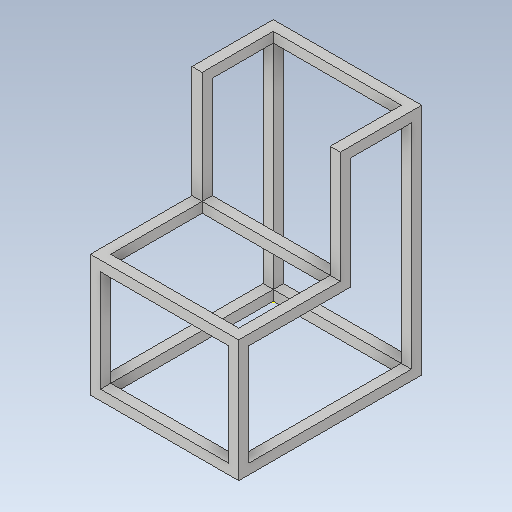
# Autodesk Inventor part: fuel tank housing
Saved by Autodesk Inventor 2020 (Build 240168000, 168)
## iProperties
Created: 2020-10-15
Part Number: fuel tank housing
Material: Generic
Document SubType Name: Modeling
Designer: nabee
Density: 1 g/cm^3
Appearance: Default
Author: nabee
Autodesk Inventor part; units mm, degrees
ref_plane "YZ Plane" through (0, 0, 0) normal (1, 0, 0) x (0, 1, 0)
ref_plane "XZ Plane" through (0, 0, 0) normal (0, 1, 0) x (-1, 0, 0)
ref_plane "XY Plane" through (0, 0, 0) normal (0, 0, 1) x (1, 0, 0)
sketch "Sketch1" plane through (0, 0, 0) normal (0, 0, 1) x (1, 0, 0)
  line L0 (0, 0) -> (220, 0)
  line L1 (220, 0) -> (220, 480)
  line L2 (220, 480) -> (0, 480)
  line L3 (0, 480) -> (0, 0)
  dimension "d0" = 480
  dimension "d1" = 220
  constraints: 8 end point, 2 parallel, 1 horizontal, 1 perpendicular
  measures "d0" distance of L2.end L0.start
  measures "d1" distance of L0.start L0.end
extrude "Extrusion1" add sketch "Sketch1" along normal blind 360
sketch "Sketch2" plane through (0, 480, 0) normal (0, 1, 0) x (1, 0, 0)
  line L0 (220, 0) -> (220, -360) projected
  line L1 (0, 0) -> (220, 0)
  line L2 (220, 0) -> (220, -160)
  line L3 (220, -160) -> (0, -160)
  line L4 (0, -160) -> (0, 0)
  line L5 (20, -20) -> (200, -20)
  line L6 (200, -20) -> (200, -140)
  line L7 (200, -140) -> (20, -140)
  line L8 (20, -140) -> (20, -20)
  line L9 (0, -360) -> (220, -360) projected
  line L10 (0, -160) -> (220, -160)
  line L11 (220, -160) -> (220, -360)
  line L12 (220, -360) -> (0, -360)
  line L13 (0, -360) -> (0, -160)
  dimension "d4" = 160
  dimension "d5" = 20
  dimension "d6" = 20
  dimension "d7" = 20
  dimension "d8" = 20
  constraints: 24 end point, 6 parallel, 3 horizontal, 3 perpendicular, 1 point on line
  measures "d4" distance of L3.end L1.start
  measures "d5" distance between parallel lines of L1 L5
  measures "d6" distance between parallel lines of L4 L8
  measures "d7" distance between parallel lines of L0 L6
  measures "d8" distance between parallel lines of L3 L7
extrude "Extrusion2" cut sketch "Sketch2" against normal blind 220 contours L0 L9 L13 L3
sketch "Sketch3" plane through (220, 0, 0) normal (1, 0, 0) x (0, 0, -1)
  line L0 (-20, 240) -> (-20, 20)
  line L1 (-20, 20) -> (-340, 20)
  line L2 (-340, 20) -> (-340, 240)
  line L3 (-160, 260) -> (-360, 260) projected
  line L4 (-360, 0) -> (-360, 260) projected
  line L5 (0, 0) -> (-360, 0) projected
  line L6 (0, 0) -> (0, 480) projected
  line L7 (-340, 240) -> (-140, 240)
  line L8 (-140, 240) -> (-140, 460)
  line L9 (-140, 460) -> (-20, 460)
  line L10 (-20, 460) -> (-20, 240)
  line L11 (-160, 480) -> (-160, 260) projected
  line L12 (0, 480) -> (-160, 480) projected
  dimension "d12" = 20
  dimension "d13" = 20
  dimension "d14" = 20
  dimension "d16" = 20
  dimension "d17" = 20
  dimension "d18" = 20
  constraints: 14 end point, 2 equal length, 2 perpendicular, 1 horizontal
  measures "d12" distance between parallel lines of L4 L2
  measures "d13" distance between parallel lines of L5 L1
  measures "d14" distance between parallel lines of L6 L0
  measures "d16" distance between parallel lines of L11 L8
  measures "d17" distance between parallel lines of L12 L9
  measures "d18" distance between parallel lines of L3 L7
extrude "Extrusion3" cut sketch "Sketch3" against normal blind 220 contours L0 L1 L2 L7 L8 L9 L10
sketch "Sketch4" plane through (0, 0, 360) normal (0, 0, 1) x (1, 0, 0)
  line L0 (20, 240) -> (200, 240)
  line L1 (200, 240) -> (200, 20)
  line L2 (200, 20) -> (20, 20)
  line L3 (20, 20) -> (20, 240)
  line L4 (220, 260) -> (0, 260) projected
  line L5 (0, 260) -> (0, 0) projected
  line L6 (0, 0) -> (220, 0) projected
  line L7 (220, 0) -> (220, 260) projected
  dimension "d21" = 20
  dimension "d22" = 20
  dimension "d23" = 20
  dimension "d24" = 20
  constraints: 8 end point, 2 parallel, 1 horizontal, 1 perpendicular
  measures "d21" distance between parallel lines of L4 L0
  measures "d22" distance between parallel lines of L5 L3
  measures "d23" distance between parallel lines of L6 L2
  measures "d24" distance between parallel lines of L7 L1
extrude "Extrusion4" cut sketch "Sketch4" against normal blind 600 contours L0 L1 L2 L3
sketch "Sketch5" plane through (0, 0, 0) normal (0, -1, 0) x (1, 0, 0)
  line L0 (200, 20) -> (200, 0) projected
  line L1 (20, 340) -> (200, 340)
  line L2 (200, 340) -> (200, 20)
  line L3 (200, 20) -> (20, 20)
  line L4 (20, 20) -> (20, 340)
  point P0 (0, 0)
  constraints: 8 end point, 2 parallel, 1 horizontal, 1 perpendicular
extrude "Extrusion5" cut sketch "Sketch5" against normal blind 900
sketch "Sketch6" plane through (0, 0, 0) normal (0, 0, -1) x (-1, 0, 0)
  line L0 (-220, 240) -> (-200, 240) projected
  line L1 (-20, 460) -> (-20, 240) projected
  line L2 (-200, 240) -> (-20, 240)
  line L3 (-20, 240) -> (-20, 460)
  line L4 (-20, 460) -> (-200, 460)
  line L5 (-200, 460) -> (-200, 240)
  point P0 (0, 0)
  constraints: 8 end point, 2 parallel, 1 horizontal, 1 perpendicular
extrude "Extrusion6" cut sketch "Sketch6" against normal blind 80
sketch "Sketch7" plane through (20, 260, 160) normal (1, 0, 0) x (0, 0, -1)
  line L0 (20, 200) -> (20, -20) projected
  line L1 (20, -20) -> (0, -20)
  line L2 (0, -20) -> (0, 0)
  line L3 (0, 0) -> (20, 0)
  line L4 (20, 0) -> (20, -20)
  point P0 (160, -260)
  constraints: 8 end point, 2 parallel, 1 horizontal, 1 perpendicular
extrude "Extrusion7" add sketch "Sketch7" along normal blind 180
sketch "Sketch8" plane through (0, 0, 0) normal (0, -1, 0) x (1, 0, 0)
  point P0 (0, 0)
sketch "Sketch9" plane through (220, 0, 0) normal (1, 0, 0) x (0, 0, -1)
  line L0 (-360, 0) -> (-360, 260) projected
  line L1 (-360, 0) -> (-360, 260)
  line L2 (-360, 260) -> (-160, 260)
  line L3 (-160, 480) -> (-20, 480) projected
  line L4 (-160, 260) -> (-160, 480)
  line L5 (-160, 480) -> (0, 480)
  line L6 (0, 480) -> (0, 0)
  line L7 (0, 0) -> (-360, 0)
  constraints: 12 end point, 4 perpendicular, 1 collinear, 1 vertical
extrude "Extrusion8" add sketch "Sketch9" along normal blind 72
sketch "Sketch10" plane through (292, 0, 0) normal (1, 0, 0) x (0, 0, -1)
  line L0 (-340, 20) -> (-340, 240) projected
  line L1 (-340, 240) -> (-340, 20)
  line L2 (-20, 20) -> (-340, 20) projected
  line L3 (-340, 20) -> (-20, 20)
  line L4 (0, 460) -> (-20, 460) projected
  line L5 (-20, 20) -> (-20, 460)
  line L6 (-20, 460) -> (-140, 460)
  line L7 (-140, 240) -> (-340, 240) projected
  line L8 (-140, 460) -> (-140, 240)
  line L9 (-140, 240) -> (-340, 240)
  point P0 (0, 0)
  constraints: 12 end point, 3 perpendicular, 2 collinear, 1 vertical
extrude "Extrusion9" cut sketch "Sketch10" against normal blind 150
sketch "Sketch11" plane through (0, 0, 360) normal (0, 0, 1) x (1, 0, 0)
  line L0 (20, 240) -> (200, 240) projected
  line L1 (292, 20) -> (200, 20) projected
  line L2 (200, 240) -> (272, 240)
  line L3 (272, 240) -> (272, 20)
  line L4 (272, 20) -> (200, 20)
  line L5 (200, 20) -> (200, 240)
  line L6 (292, 260) -> (292, 0) projected
  point P0 (0, 0)
  dimension "d37" = 20
  constraints: 8 end point, 2 parallel, 1 horizontal, 1 perpendicular, 1 point on line
  measures "d37" distance between parallel lines of L6 L3
extrude "Extrusion10" cut sketch "Sketch11" against normal blind 900
sketch "Sketch12" plane through (0, 260, 0) normal (0, 1, 0) x (1, 0, 0)
  line L0 (200, -340) -> (200, -160) projected
  line L1 (200, -160) -> (272, -160)
  line L2 (272, -160) -> (272, -340)
  line L3 (272, -340) -> (200, -340)
  line L4 (200, -340) -> (200, -160)
  line L5 (292, -160) -> (292, -360) projected
  point P0 (0, 0)
  dimension "d40" = 20
  constraints: 8 end point, 2 parallel, 1 horizontal, 1 perpendicular
  measures "d40" distance between parallel lines of L5 L2
extrude "Extrusion11" cut sketch "Sketch12" against normal blind 900
sketch "Sketch13" plane through (20, 260, 160) normal (0, 0, 1) x (1, 0, 0)
  line L0 (180, 200) -> (0, 200) projected
  line L1 (252, 0) -> (272, 0) projected
  line L2 (180, 200) -> (252, 200)
  line L3 (252, 200) -> (252, 0)
  line L4 (252, 0) -> (180, 0)
  line L5 (180, 0) -> (180, 200)
  point P0 (-20, -260)
  constraints: 8 end point, 2 parallel, 1 horizontal, 1 perpendicular
extrude "Extrusion12" cut sketch "Sketch13" against normal blind 900
sketch "Sketch14" plane through (0, 480, 160) normal (0, 1, 0) x (1, 0, 0)
  line L0 (200, 140) -> (200, 0) projected
  line L1 (292, 140) -> (272, 140) projected
  line L2 (200, 0) -> (272, 0)
  line L3 (272, 0) -> (272, 140)
  line L4 (272, 140) -> (200, 140)
  line L5 (200, 140) -> (200, 0)
  point P0 (0, 160)
  constraints: 8 end point, 2 parallel, 1 horizontal, 1 perpendicular
extrude "Extrusion13" cut sketch "Sketch14" against normal blind 900
sketch "Sketch15" plane through (200, 240, 140) normal (1, 0, 0) x (0, 0, -1)
  line L0 (-220, 20) -> (-20, 20) projected
  line L1 (0, 0) -> (-200, 0) projected
  line L2 (-20, 20) -> (0, 20)
  line L3 (0, 20) -> (0, 0)
  line L4 (0, 0) -> (-20, 0)
  line L5 (-20, 0) -> (-20, 20)
  point P0 (140, -240)
  constraints: 8 end point, 2 parallel, 1 horizontal, 1 perpendicular
extrude "Extrusion14" add sketch "Sketch15" along normal up to next
sketch "Sketch16" plane through (200, 240, 0) normal (-1, 0, 0) x (0, 0, 1)
  line L0 (20, 20) -> (0, 20) projected
  line L1 (20, 0) -> (20, -220) projected
  line L2 (0, 20) -> (20, 20)
  line L3 (20, 20) -> (20, 0)
  line L4 (20, 0) -> (0, 0)
  line L5 (0, 0) -> (0, 20)
  point P0 (0, -240)
  constraints: 8 end point, 2 parallel, 1 horizontal, 1 perpendicular
extrude "Extrusion15" cut sketch "Sketch16" against normal up to surface (72 mm away) from surface at 0
sketch "Sketch17" plane through (0, 0, 0) normal (0, -1, 0) x (1, 0, 0)
  line L0 (292, 360) -> (0, 360) projected
  line L1 (292, 360) -> (292, 0) projected
  line L2 (0, 360) -> (292, 360)
  line L3 (292, 360) -> (292, 0)
  line L4 (292, 0) -> (0, 0)
  line L5 (0, 0) -> (0, 360)
  point P0 (0, 0)
  constraints: 8 end point, 2 parallel, 1 horizontal, 1 perpendicular
extrude "Extrusion16" cut sketch "Sketch17" against normal blind 20
sketch "Sketch18" plane through (0, 0, 360) normal (0, 0, 1) x (1, 0, 0)
  line L0 (0, 20) -> (292, 20)
  line L1 (292, 20) -> (292, 40)
  line L2 (292, 40) -> (0, 40)
  line L3 (0, 40) -> (0, 20)
  point P0 (0, 0)
  dimension "d53" = 20
  constraints: 8 end point, 2 parallel, 1 horizontal, 1 perpendicular
  measures "d53" distance of L2.end L0.start
extrude "Extrusion17" add sketch "Sketch18" against normal blind 360
sketch "Sketch19" plane through (0, 20, 0) normal (0, -1, 0) x (1, 0, 0)
  line L0 (20, 360) -> (20, 340) projected
  line L1 (20, 340) -> (272, 340)
  line L2 (272, 340) -> (272, 20)
  line L3 (272, 20) -> (20, 20)
  line L4 (20, 20) -> (20, 340)
  point P0 (0, 0)
  constraints: 8 end point, 2 parallel, 1 horizontal, 1 perpendicular
extrude "Extrusion18" cut sketch "Sketch19" against normal blind 60
body "Solid1"
